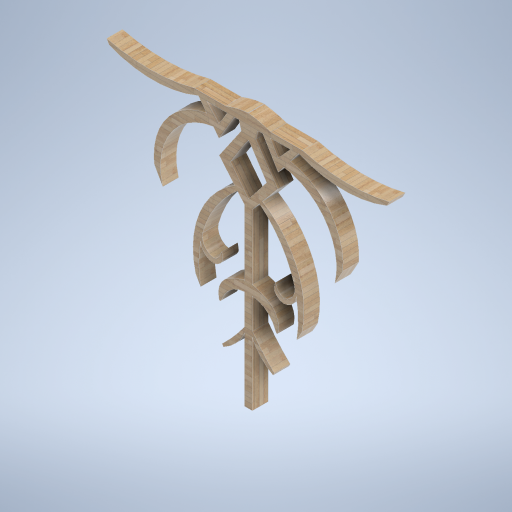
# Autodesk Inventor part: side_art_frame_01
Saved by Autodesk Inventor 2024.2 (Build 282272000, 272)
## iProperties
Created: 2024-05-25
Part Number: side_art_frame_01
Material: Wood (Maple)
Document SubType Name: Modeling
Designer: LOSTER_1
Density: 0.67 g/cm^3
Appearance: Natural Maple - Glossy Dark Tint
Author: LOSTER_1
Autodesk Inventor part; units mm, degrees
ref_plane "YZ Plane" through (0, 0, 0) normal (1, 0, 0) x (0, 1, 0)
ref_plane "XZ Plane" through (0, 0, 0) normal (0, 1, 0) x (-1, 0, 0)
ref_plane "XY Plane" through (0, 0, 0) normal (0, 0, 1) x (1, 0, 0)
sketch "Sketch1" plane through (0, 0, 0) normal (0, 0, 1) x (1, 0, 0)
  line L0 (-3091.9119, -1486.6616) -> (-1314.1662, 1691.7457)
  line L1 (-3091.9119, -1538.7933) -> (-3091.9119, -1486.6616)
  line L2 (-3191.9119, -1538.7933) -> (-3091.9119, -1538.7933)
  line L3 (-1314.1662, 1691.7457) -> (-3086.603, 1689.7264)
  line L4 (-3188.5143, -1502.5516) -> (-4974.1409, 1689.7264)
  line L5 (-3188.5132, -1538.7933) -> (-3188.5143, -1502.5516)
  line L6 (-3086.603, 1689.7264) -> (-4974.1409, 1689.7264)
  line L7 (-3086.603, 1689.7264) -> (1064.8557, 1689.7264) construction
  point P0 (0, 0)
  dimension "d0" = 180
  constraints: 16 end point, 1 horizontal, 1 point on line
  measures "d0" angle of L6 L7
extrude "Extrusion1" add sketch "Sketch1" along normal blind 200
sketch "Sketch2" plane through (0, 0, 0) normal (0, 0, -1) x (-1, 0, 0)
  line L0 (3188.5143, -1502.5516) -> (3188.5132, -1538.7933) projected
  line L1 (4974.1409, 1689.7264) -> (3188.5143, -1502.5516) projected
  line L2 (3086.603, 1689.7264) -> (4974.1409, 1689.7264) projected
  line L3 (1314.1662, 1691.7457) -> (3086.603, 1689.7264) projected
  line L4 (3091.9119, -1486.6616) -> (1314.1662, 1691.7457) projected
  line L5 (3091.9119, -1538.7933) -> (3091.9119, -1486.6616) projected
  line L6 (3188.5132, -1538.7933) -> (3091.9119, -1538.7933) projected
  line L7 (3188.5143, -1502.5516) -> (3188.5132, -1538.7933) projected
  line L8 (3188.5132, -1538.7933) -> (3091.9119, -1538.7933)
  line L9 (3091.9119, -1538.7933) -> (3091.9119, -738.7933)
  arc A0 (2830.6682, -1019.5876) -> (3091.9119, -738.7933) centre (2545.0491, -491.9308) ccw
  line L10 (3091.9119, -738.7933) -> (3091.9119, -668.5524)
  line L11 (3091.9119, -1486.6616) -> (1314.1662, 1691.7457) projected
  line L12 (3140.2126, -1538.7933) -> (3140.2126, -1771.7265)
  line L13 (3091.9119, -738.7933) -> (3091.9119, 661.2067)
  line L14 (3091.9119, 661.2067) -> (2770.5181, 1044.2289)
  line L15 (3091.9119, 811.5722) -> (2910.8944, 1044.2289)
  line L16 (2910.8944, 1044.2289) -> (3091.9119, 1327.5071)
  arc A1 (3001.4031, 769.0708) -> (2532.0152, -485.63) centre (3848.9496, -263.1495) ccw
  arc A2 (2965.7402, 811.5722) -> (2465.9601, -367.5309) centre (3540.5562, -127.5431) ccw
  arc A3 (2564.3939, 102.5421) -> (2698.966, -113.5984) centre (2723.5279, 51.6576) ccw
  arc A4 (2698.966, -113.5984) -> (2791.5063, -19.2445) centre (2672.2057, 5.2052) ccw
  arc A5 (2803.0097, 5.2052) -> (2791.5063, -19.2445) centre (2834.0555, -24.3325) ccw
  arc A6 (2814.0726, -88.7508) -> (2803.0097, 5.2052) centre (2565.5117, -70.3883) ccw
  arc A7 (2698.966, -171.4535) -> (2814.0726, -88.7508) centre (2682.1111, -26.5401) ccw
  arc A8 (2536.7293, -14.3693) -> (2698.966, -171.4535) centre (2705.1387, -2.7572) ccw
  arc A9 (3091.9119, -286.7362) -> (2802.6332, -512.5472) centre (3119.1212, -619.791) ccw
  line L17 (3001.4031, 1622.7638) -> (2767.2375, 1228.8671)
  line L18 (2767.2375, 1228.8671) -> (2460.7681, 1622.7638)
  line L19 (2460.7681, 1622.7638) -> (3001.4031, 1622.7638)
  line L20 (2767.2375, 1384.92) -> (2868.6354, 1555.4844)
  line L21 (2868.6354, 1555.4844) -> (2614.0028, 1555.4844)
  line L22 (2614.0028, 1555.4844) -> (2767.2375, 1384.92)
  arc A10 (2695.7962, 1320.6887) -> (2050.6798, 374.943) centre (2801.4572, 555.7171) ccw
  arc A11 (2614.0028, 1425.8155) -> (1949.5694, 555.7171) centre (2750.2147, 633.06) ccw
  line L23 (2770.5181, 1044.2289) -> (3049.1233, 1448.187)
  line L24 (3049.1233, 1448.187) -> (3001.4031, 1622.7638)
  arc A12 (2781.4228, -543.6749) -> (2802.6332, -512.5472) centre (2736.101, -490.0023) ccw
  arc A13 (2767.2375, -520.4351) -> (2781.4228, -543.6749) centre (2794.3216, -519.8525) ccw
  arc A14 (2900.2757, -237.1487) -> (2767.2375, -520.4351) centre (3006.8658, -460.0882) ccw
  arc A15 (3091.9119, -159.8121) -> (2900.2757, -237.1487) centre (3342.9537, -1057.9822) ccw
  line L25 (3188.5132, -1538.7933) -> (3188.5132, -738.7933)
  arc A16 (3188.5132, -738.7933) -> (3449.7569, -1019.5876) centre (3735.376, -491.9308) ccw
  line L26 (3188.5132, -738.7933) -> (3188.5132, 661.2067)
  line L27 (3188.5132, 661.2067) -> (3509.907, 1044.2289)
  line L28 (3188.5132, 811.5722) -> (3369.5307, 1044.2289)
  line L29 (3369.5307, 1044.2289) -> (3188.5132, 1327.5071)
  arc A17 (3748.4099, -485.63) -> (3279.022, 769.0708) centre (2431.4755, -263.1495) ccw
  arc A18 (3814.465, -367.5309) -> (3314.6849, 811.5722) centre (2739.8689, -127.5431) ccw
  arc A19 (3581.4591, -113.5984) -> (3716.0312, 102.5421) centre (3556.8972, 51.6576) ccw
  arc A20 (3488.9188, -19.2445) -> (3581.4591, -113.5984) centre (3608.2194, 5.2052) ccw
  arc A21 (3488.9188, -19.2445) -> (3477.4154, 5.2052) centre (3446.3696, -24.3325) ccw
  arc A22 (3477.4154, 5.2052) -> (3466.3525, -88.7508) centre (3714.9134, -70.3883) ccw
  arc A23 (3466.3525, -88.7508) -> (3581.4591, -171.4535) centre (3598.314, -26.5401) ccw
  arc A24 (3581.4591, -171.4535) -> (3743.6958, -14.3693) centre (3575.2864, -2.7572) ccw
  arc A25 (3477.7919, -512.5472) -> (3188.5132, -286.7362) centre (3161.3039, -619.791) ccw
  line L30 (3279.022, 1622.7638) -> (3513.1876, 1228.8671)
  line L31 (3513.1876, 1228.8671) -> (3819.657, 1622.7638)
  line L32 (3819.657, 1622.7638) -> (3279.022, 1622.7638)
  line L33 (3513.1876, 1384.92) -> (3411.7897, 1555.4844)
  line L34 (3411.7897, 1555.4844) -> (3666.4223, 1555.4844)
  line L35 (3666.4223, 1555.4844) -> (3513.1876, 1384.92)
  arc A26 (4229.7453, 374.943) -> (3584.6289, 1320.6887) centre (3478.9679, 555.7171) ccw
  arc A27 (4330.8558, 555.7171) -> (3666.4223, 1425.8155) centre (3530.2104, 633.06) ccw
  line L36 (3509.907, 1044.2289) -> (3231.3018, 1448.187)
  line L37 (3231.3018, 1448.187) -> (3279.022, 1622.7638)
  arc A28 (3477.7919, -512.5472) -> (3499.0023, -543.6749) centre (3544.3241, -490.0023) ccw
  arc A29 (3499.0023, -543.6749) -> (3513.1876, -520.4351) centre (3486.1035, -519.8525) ccw
  arc A30 (3513.1876, -520.4351) -> (3380.1494, -237.1487) centre (3273.5593, -460.0882) ccw
  arc A31 (3380.1494, -237.1487) -> (3188.5132, -159.8121) centre (2937.4714, -1057.9822) ccw
  arc A32 (2813.9776, -989.7466) -> (3091.9119, -668.5524) centre (1245.8024, 648.0673) ccw
  arc A33 (3188.5132, -668.5524) -> (3466.4475, -989.7466) centre (5034.6227, 648.0673) ccw
  line L38 (3188.5132, 811.5722) -> (3140.2126, 749.4927)
  line L39 (3091.9119, 811.5722) -> (3140.2126, 749.4927)
  line L40 (3188.5132, 1327.5071) -> (3140.2126, 1394.0359)
  line L41 (3140.2126, 1394.0359) -> (3091.9119, 1327.5071)
  line L42 (4974.1409, 1689.7264) -> (3188.5143, -1502.5516) projected
  arc A34 (3819.657, 1622.7638) -> (4930.1634, 1611.1051) centre (4397.1884, 3738.9435) ccw
  arc A35 (3773.7375, 1563.7448) -> (4899.0515, 1555.4844) centre (4346.2773, 2905.9325) ccw
  arc A36 (1360.72, 1608.5128) -> (2460.7681, 1622.7638) centre (1883.2367, 3738.9435) ccw
  arc A37 (1393.0117, 1550.7789) -> (2506.6876, 1563.7448) centre (1934.1479, 2905.9325) ccw
  line L43 (3188.5143, -1502.5516) -> (4974.1409, 1689.7264)
  line L44 (4974.1409, 1689.7264) -> (1314.1662, 1691.7457)
  line L45 (1314.1662, 1691.7457) -> (3091.9119, -1486.6616)
  line L46 (3279.022, 1622.7638) -> (3144.1535, 1690.736)
  line L47 (3001.4031, 1622.7638) -> (3144.1535, 1690.736)
  arc A38 (3427.51, -1006.9245) -> (3456.6186, -1023.2446) centre (3735.376, -491.9308) ccw
  line L48 (3464.2808, -987.6692) -> (3464.2808, -987.6692)
  line L49 (3472.3566, -995.1087) -> (3451.0443, -974.8581)
  arc A39 (3807.9007, -395.2353) -> (3828.554, -292.2114) centre (2739.8689, -127.5431) ccw
  arc A40 (3744.239, -509.0473) -> (3761.6531, -383.3216) centre (2431.4755, -263.1495) ccw
  arc A41 (4327.6537, 533.9602) -> (4334.561, 627.1442) centre (3487.8698, 643.0578) ccw
  arc A42 (4221.8358, 344.7827) -> (4244.1993, 451.9539) centre (3478.9679, 555.7171) ccw
  point P0 (0, 0)
  point P1 (1350.2617, 1611.1051)
  point P2 (1381.3736, 1555.4844)
  point P3 (1949.5694, 555.7171)
  point P4 (2532.0152, -485.63)
  point P5 (2813.9776, -989.7466)
  point P6 (2561.0883, 90.7249)
  point P7 (2050.6798, 374.943)
  point P8 (3142.0332, 1689.7264)
  point P9 (4930.1634, 1611.1051)
  point P10 (3146.1569, 1689.7264)
  point P11 (3807.9007, -395.2353)
  point P12 (4221.8358, 344.7827)
  point P13 (3719.3368, 90.7249)
  point P14 (3188.5132, -668.5524)
  point P15 (3748.4099, -485.63)
  point P16 (3456.6186, -1023.2446)
  point P17 (3449.7569, -1019.5876)
  dimension "d4" = 800
  dimension "d7" = 600
  dimension "d9" = 1400
  dimension "d10" = 500
  dimension "d11" = 140
  constraints: 102 point on circle, 80 end point, 60 symmetric about line, 43 centre point, 24 point on line, 4 concentric, 3 midpoint, 2 collinear, 2 parallel, 2 tangent, 1 perpendicular, 1 vertical, 27 other
  measures "d4" distance of L5.start L9.end
  measures "d7" radius of A0
  measures "d9" distance of L9.end L13.end
  measures "d10" distance of L13.end L14.end
  measures "d11" angle of L14 L13
extrude "Extrusion2" cut sketch "Sketch2" against normal through all contours L25 A16 A38 L1 | L49 A33 L26 A25 A28 A29 A30 A31 L27 A17 A19 A20 A21 A22 A23 A24 A40 L1 | L4 A0 L9 | A39 A18 L27 L36 L37 L30 L31 A26 A42 L1 | L4 A1 A8 A7 A6 A5 A4 A3 L14 L13 A15 A14 A13 A12 A9 A32 | A41 A27 L31 A35 L1 | L4 A10 L18 L17 L24 L23 L14 A2 | A34 L32 L46 L2 L1 | L4 A37 L18 A11 | L47 L19 A36 L4 L3 L2 | L15 L16 L41 L40 L29 L28 L38 L39 | L22 L21 L20 | L33 L34 L35
sketch "Sketch3" plane through (0, 0, 200) normal (0, 0, 1) x (1, 0, 0)
  line L0 (-3001.4031, 1622.7638) -> (-3142.0332, 1689.7264) projected
  line L1 (-3146.1569, 1689.7264) -> (-3279.022, 1622.7638) projected
  line L2 (-2460.7681, 1622.7638) -> (-3001.4031, 1622.7638) projected
  line L3 (-3279.022, 1622.7638) -> (-3819.657, 1622.7638) projected
  arc A0 (-2858.3401, 1622.7638) -> (-3146.1569, 1689.7264) centre (-3295.5109, 395.7514) ccw
  line L4 (-3819.657, 1622.7638) -> (-3279.022, 1622.7638) projected
  arc A1 (-3146.1569, 1689.7264) -> (-3427.0308, 1622.7638) centre (-3072.1927, 756.9406) ccw
  line L5 (-3001.4031, 1622.7638) -> (-2767.2375, 1228.8671) projected
  line L6 (-3049.1233, 1448.187) -> (-3001.4031, 1622.7638) projected
  line L7 (-3279.022, 1622.7638) -> (-3231.3018, 1448.187) projected
  line L8 (-3513.1876, 1228.8671) -> (-3279.022, 1622.7638) projected
  line L9 (-2868.6354, 1555.4844) -> (-2614.0028, 1555.4844) projected
  line L10 (-3666.4223, 1555.4844) -> (-3411.7897, 1555.4844) projected
  line L11 (-2868.6354, 1555.4844) -> (-2767.2375, 1384.92) projected
  line L12 (-2868.6354, 1555.4844) -> (-3411.7897, 1555.4844)
  point P0 (0, 0)
  point P1 (-3140.6812, 1689.0826)
  point P2 (-3319.0186, 1555.4844)
  point P3 (-3260.6313, 1555.4844)
  point P4 (-3019.7938, 1555.4844)
  point P5 (-2961.4065, 1555.4844)
  constraints: 4 point on circle, 2 centre point, 2 end point, 2 point on line, 1 horizontal
extrude "Extrusion3" add sketch "Sketch3" against normal blind 200 contours L0 A0 L2 | L5 L12 L6 | L1 L3 A1 | L12 L8 L7
ref_plane "Work Plane1" through (0, 0, 100) normal (0, 0, -1) x (-1, 0, 0)
sketch "Sketch4" plane through (0, 0, 100) normal (0, 0, -1) x (-1, 0, 0)
  line L0 (2767.2375, 1384.92) -> (2614.0028, 1555.4844) projected
  line L1 (2614.0028, 1555.4844) -> (2868.6354, 1555.4844) projected
  line L2 (2868.6354, 1555.4844) -> (2767.2375, 1384.92) projected
  line L3 (3140.2126, 1394.0359) -> (3188.5132, 1327.5071) projected
  line L4 (3188.5132, 1327.5071) -> (3369.5307, 1044.2289) projected
  line L5 (3369.5307, 1044.2289) -> (3140.2126, 749.4927) projected
  line L6 (3140.2126, 749.4927) -> (2910.8944, 1044.2289) projected
  line L7 (2910.8944, 1044.2289) -> (3091.9119, 1327.5071) projected
  line L8 (3091.9119, 1327.5071) -> (3140.2126, 1394.0359) projected
  arc A0 (3773.7375, 1563.7448) -> (4899.0515, 1555.4844) centre (4346.2773, 2905.9325) ccw projected
  line L9 (4930.1634, 1611.1051) -> (4899.0515, 1555.4844) projected
  arc A1 (3819.657, 1622.7638) -> (4930.1634, 1611.1051) centre (4397.1884, 3738.9435) ccw projected
  line L10 (3819.657, 1622.7638) -> (3427.0308, 1622.7638) projected
  arc A2 (3427.0308, 1622.7638) -> (3146.1569, 1689.7264) centre (3072.1927, 756.9406) ccw projected
  line L11 (3142.0332, 1689.7264) -> (3146.1569, 1689.7264) projected
  line L12 (3142.0332, 1689.7264) -> (3140.6812, 1689.0826) projected
  arc A3 (3140.6812, 1689.0826) -> (2858.3401, 1622.7638) centre (3295.5109, 395.7514) ccw projected
  line L13 (2858.3401, 1622.7638) -> (2460.7681, 1622.7638) projected
  arc A4 (1360.72, 1608.5128) -> (2460.7681, 1622.7638) centre (1883.2367, 3738.9435) ccw projected
  line L14 (1393.0117, 1550.7789) -> (1360.72, 1608.5128) projected
  arc A5 (1393.0117, 1550.7789) -> (2506.6876, 1563.7448) centre (1934.1479, 2905.9325) ccw projected
  line L15 (2506.6876, 1563.7448) -> (2614.0028, 1425.8155) projected
  arc A6 (2614.0028, 1425.8155) -> (1949.5694, 555.7171) centre (2750.2147, 633.06) ccw projected
  line L16 (2050.6798, 374.943) -> (1949.5694, 555.7171) projected
  arc A7 (2695.7962, 1320.6887) -> (2050.6798, 374.943) centre (2801.4572, 555.7171) ccw projected
  line L17 (2695.7962, 1320.6887) -> (2767.2375, 1228.8671) projected
  line L18 (2767.2375, 1228.8671) -> (2961.4065, 1555.4844) projected
  line L19 (2961.4065, 1555.4844) -> (3019.7938, 1555.4844) projected
  line L20 (3019.7938, 1555.4844) -> (3049.1233, 1448.187) projected
  line L21 (3049.1233, 1448.187) -> (2770.5181, 1044.2289) projected
  line L22 (2770.5181, 1044.2289) -> (2965.7402, 811.5722) projected
  arc A8 (2965.7402, 811.5722) -> (2465.9601, -367.5309) centre (3540.5562, -127.5431) ccw projected
  line L23 (2532.0152, -485.63) -> (2465.9601, -367.5309) projected
  arc A9 (2536.7293, -14.3693) -> (2532.0152, -485.63) centre (3848.9496, -263.1495) ccw projected
  arc A10 (2536.7293, -14.3693) -> (2698.966, -171.4535) centre (2705.1387, -2.7572) ccw projected
  arc A11 (2698.966, -171.4535) -> (2814.0726, -88.7508) centre (2682.1111, -26.5401) ccw projected
  arc A12 (2814.0726, -88.7508) -> (2803.0097, 5.2052) centre (2565.5117, -70.3883) ccw projected
  arc A13 (2803.0097, 5.2052) -> (2791.5063, -19.2445) centre (2834.0555, -24.3325) ccw projected
  arc A14 (2698.966, -113.5984) -> (2791.5063, -19.2445) centre (2672.2057, 5.2052) ccw projected
  arc A15 (2561.0883, 90.7249) -> (2698.966, -113.5984) centre (2723.5279, 51.6576) ccw projected
  arc A16 (3001.4031, 769.0708) -> (2561.0883, 90.7249) centre (3848.9496, -263.1495) ccw projected
  line L24 (3001.4031, 769.0708) -> (3091.9119, 661.2067) projected
  line L25 (3091.9119, 661.2067) -> (3091.9119, -159.8121) projected
  arc A17 (3091.9119, -159.8121) -> (2900.2757, -237.1487) centre (3342.9537, -1057.9822) ccw projected
  arc A18 (2900.2757, -237.1487) -> (2767.2375, -520.4351) centre (3006.8658, -460.0882) ccw projected
  arc A19 (2767.2375, -520.4351) -> (2781.4228, -543.6749) centre (2794.3216, -519.8525) ccw projected
  arc A20 (2781.4228, -543.6749) -> (2802.6332, -512.5472) centre (2736.101, -490.0023) ccw projected
  arc A21 (3091.9119, -286.7362) -> (2802.6332, -512.5472) centre (3119.1212, -619.791) ccw projected
  line L26 (3091.9119, -286.7362) -> (3091.9119, -668.5524) projected
  arc A22 (2813.9776, -989.7466) -> (3091.9119, -668.5524) centre (1245.8024, 648.0673) ccw projected
  line L27 (2830.6682, -1019.5876) -> (2813.9776, -989.7466) projected
  arc A23 (2830.6682, -1019.5876) -> (3091.9119, -738.7933) centre (2545.0491, -491.9308) ccw projected
  line L28 (3091.9119, -1538.7933) -> (3091.9119, -738.7933) projected
  line L29 (3188.5132, -1538.7933) -> (3091.9119, -1538.7933) projected
  line L30 (3188.5132, -1538.7933) -> (3188.5132, -738.7933) projected
  arc A24 (3188.5132, -738.7933) -> (3456.6186, -1023.2446) centre (3735.376, -491.9308) ccw projected
  line L31 (3472.3566, -995.1087) -> (3456.6186, -1023.2446) projected
  line L32 (3472.3566, -995.1087) -> (3451.0443, -974.8581) projected
  arc A25 (3188.5132, -668.5524) -> (3451.0443, -974.8581) centre (5034.6227, 648.0673) ccw projected
  line L33 (3188.5132, -668.5524) -> (3188.5132, -286.7362) projected
  arc A26 (3477.7919, -512.5472) -> (3188.5132, -286.7362) centre (3161.3039, -619.791) ccw projected
  arc A27 (3477.7919, -512.5472) -> (3499.0023, -543.6749) centre (3544.3241, -490.0023) ccw projected
  arc A28 (3499.0023, -543.6749) -> (3513.1876, -520.4351) centre (3486.1035, -519.8525) ccw projected
  arc A29 (3513.1876, -520.4351) -> (3380.1494, -237.1487) centre (3273.5593, -460.0882) ccw projected
  arc A30 (3380.1494, -237.1487) -> (3188.5132, -159.8121) centre (2937.4714, -1057.9822) ccw projected
  line L34 (3188.5132, -159.8121) -> (3188.5132, 661.2067) projected
  line L35 (3188.5132, 661.2067) -> (3279.022, 769.0708) projected
  arc A31 (3719.3368, 90.7249) -> (3279.022, 769.0708) centre (2431.4755, -263.1495) ccw projected
  arc A32 (3581.4591, -113.5984) -> (3719.3368, 90.7249) centre (3556.8972, 51.6576) ccw projected
  arc A33 (3488.9188, -19.2445) -> (3581.4591, -113.5984) centre (3608.2194, 5.2052) ccw projected
  arc A34 (3488.9188, -19.2445) -> (3477.4154, 5.2052) centre (3446.3696, -24.3325) ccw projected
  arc A35 (3477.4154, 5.2052) -> (3466.3525, -88.7508) centre (3714.9134, -70.3883) ccw projected
  arc A36 (3466.3525, -88.7508) -> (3581.4591, -171.4535) centre (3598.314, -26.5401) ccw projected
  arc A37 (3581.4591, -171.4535) -> (3743.6958, -14.3693) centre (3575.2864, -2.7572) ccw projected
  arc A38 (3744.239, -509.0473) -> (3743.6958, -14.3693) centre (2431.4755, -263.1495) ccw projected
  line L36 (3807.9007, -395.2353) -> (3744.239, -509.0473) projected
  arc A39 (3807.9007, -395.2353) -> (3314.6849, 811.5722) centre (2739.8689, -127.5431) ccw projected
  line L37 (3314.6849, 811.5722) -> (3509.907, 1044.2289) projected
  line L38 (3509.907, 1044.2289) -> (3231.3018, 1448.187) projected
  line L39 (3231.3018, 1448.187) -> (3260.6313, 1555.4844) projected
  line L40 (3260.6313, 1555.4844) -> (3319.0186, 1555.4844) projected
  line L41 (3319.0186, 1555.4844) -> (3513.1876, 1228.8671) projected
  line L42 (3513.1876, 1228.8671) -> (3584.6289, 1320.6887) projected
  arc A40 (4221.8358, 344.7827) -> (3584.6289, 1320.6887) centre (3478.9679, 555.7171) ccw projected
  line L43 (4327.6537, 533.9602) -> (4221.8358, 344.7827) projected
  arc A41 (4327.6537, 533.9602) -> (4334.561, 627.1442) centre (3487.8698, 643.0578) ccw projected
  arc A42 (4334.561, 627.1442) -> (3666.4223, 1425.8155) centre (3530.2104, 633.06) ccw projected
  line L44 (3666.4223, 1425.8155) -> (3773.7375, 1563.7448) projected
  line L45 (3666.4223, 1555.4844) -> (3513.1876, 1384.92) projected
  line L46 (3513.1876, 1384.92) -> (3411.7897, 1555.4844) projected
  line L47 (3411.7897, 1555.4844) -> (3666.4223, 1555.4844) projected
  line L48 (1314.1662, 1691.7457) -> (3086.603, 1689.7264) projected
  line L49 (3091.9119, -1486.6616) -> (1314.1662, 1691.7457) projected
  line L50 (3086.603, 1689.7264) -> (4974.1409, 1689.7264) projected
  line L51 (3188.5143, -1502.5516) -> (4974.1409, 1689.7264) projected
  line L52 (3091.9119, -1538.7933) -> (3091.9119, -1486.6616) projected
  line L53 (3191.9119, -1538.7933) -> (3091.9119, -1538.7933) projected
  line L54 (3188.5132, -1538.7933) -> (3188.5143, -1502.5516) projected
  point P0 (0, 0)
  constraints: 2 other
body "Solid1"
